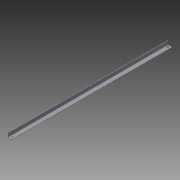
# Autodesk Inventor part: .05 in Aluminum Angle (19 in)
Saved by Autodesk Inventor 2014 (Build 180170000, 170)
## iProperties
Created: 2014-01-05
Part Number: .05 in Aluminum Angle (19 in)
Material: Generic
Document SubType Name: Modeling
Designer: Michael
Density: 1 g/cm^3
Appearance: Default
Author: Michael
Autodesk Inventor part; units mm, degrees
ref_plane "YZ Plane" through (0, 0, 0) normal (1, 0, 0) x (0, 1, 0)
ref_plane "XZ Plane" through (0, 0, 0) normal (0, 1, 0) x (-1, 0, 0)
ref_plane "XY Plane" through (0, 0, 0) normal (0, 0, 1) x (1, 0, 0)
sketch "Sketch1" plane through (0, 0, 0) normal (0, 0, 1) x (1, 0, 0)
  line L0 (0, 0) -> (12.7, 0)
  line L1 (12.7, 0) -> (12.7, 1.27)
  line L2 (12.7, 1.27) -> (1.27, 1.27)
  line L3 (1.27, 1.27) -> (1.27, 12.7)
  line L4 (1.27, 12.7) -> (0, 12.7)
  line L5 (0, 12.7) -> (0, 0)
  dimension "d0" = 12.7
  dimension "d1" = 1.27
  constraints: 12 end point, 5 perpendicular, 2 parallel, 1 horizontal
  measures "d0" distance of L0.start L0.end
  measures "d1" distance of L0.end L1.end
extrude "Extrusion1" add sketch "Sketch1" along normal blind 482.6
fillet "Fillet1" radius 1.27 4 edges at (12.7, 1.27, 241.3) (1.27, 1.27, 241.3) (1.27, 12.7, 241.3) (0, 0, 241.3)
sketch "Sketch2" plane through (2.54, 1.27, 482.6) normal (0, 1, 0) x (1, 0, 0)
  line L0 (0, 0) -> (0, 482.6) projected
  line L1 (8.89, 482.6) -> (8.89, 0) projected
  line L2 (8.89, 482.6) -> (0, 482.6) projected
  circle A0 centre (3.81, 476.25) radius 2.4892
  line L3 (-2.54, 482.6) -> (-2.54, 0) projected
  line L4 (8.89, 241.3) -> (0, 241.3) construction
  circle A1 centre (3.81, 6.35) radius 2.4892
  dimension "d6" = 4.9784
  dimension "d7" = 6.35
  dimension "d8" = 6.35
  constraints: 2 centre point, 2 end point, 2 midpoint, 1 symmetric about line, 1 other
  measures "d6" diameter of A0
  measures "d7" distance from line of L2 A0.centre
  measures "d8" distance from line of L3 A0.centre
extrude "Extrusion2" cut sketch "Sketch2" against normal blind 25.4
equation "\"d8\" = d7"
body "Solid1"
